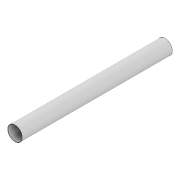
# Autodesk Inventor part: Shaft bushing lon ø14
Saved by Autodesk Inventor 2021 (Build 250183000, 183)
## iProperties
Created: 2020-11-04
Part Number: Shaft bushing lon ø14
Material: Generic
Document SubType Name: Modeling
Designer: Alfred Brauner
Density: 1 g/cm^3
Appearance: Default
Author: Alfred Brauner
Autodesk Inventor part; units mm, degrees
ref_plane "YZ Plane" through (0, 0, 0) normal (1, 0, 0) x (0, 1, 0)
ref_plane "XZ Plane" through (0, 0, 0) normal (0, 1, 0) x (-1, 0, 0)
ref_plane "XY Plane" through (0, 0, 0) normal (0, 0, 1) x (1, 0, 0)
sketch "Sketch1" plane through (0, 0, 0) normal (0, 0, 1) x (1, 0, 0)
  circle A0 centre (0, 0) radius 6
  circle A1 centre (0, 0) radius 7
  dimension "d0" = 12
  dimension "d1" = 14
  constraints: 2 centre point, 2 coincident
  measures "d0" diameter of A0
  measures "d1" diameter of A1
extrude "Extrusion1" add sketch "Sketch1" against normal mid plane 143.6
chamfer "Chamfer1" distance 0.1 angle 45 4 edges at (-6, 0, 71.8) (-7, 0, 71.8) (-7, 0, -71.8) (-6, 0, -71.8)
sketch "Sketch2" plane through (0, 0, 71.8) normal (0, 0, 1) x (1, 0, 0)
  circle A0 centre (0, 0) radius 6.5
  circle A1 centre (0, 0) radius 6
  dimension "d7" = 13
  dimension "d8" = 12
  constraints: 2 centre point, 2 coincident
  measures "d7" diameter of A0
  measures "d8" diameter of A1
extrude "Extrusion2" cut sketch "Sketch2" against normal blind 20
sketch "Sketch3" plane through (0, 0, -71.8) normal (0, 0, -1) x (-1, 0, 0)
  circle A0 centre (0, 0) radius 6.5
  dimension "d11" = 13
  constraints: 1 centre point, 1 coincident
  measures "d11" diameter of A0
extrude "Extrusion3" cut sketch "Sketch3" against normal blind 20
body "Solid1"
